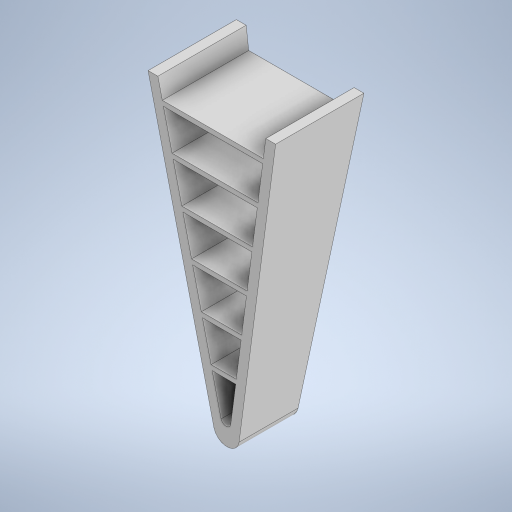
# Autodesk Inventor part: finley_gripper_60
Saved by Autodesk Inventor 2024 (Build 280153000, 153)
## iProperties
Created: 2024-09-23
Part Number: finley_gripper_60
Material: 一般
Document SubType Name: Modeling
Designer: 1412z
Density: 1 g/cm^3
Appearance: 既定
Author: 1412z
Autodesk Inventor part; units mm, degrees
ref_plane "YZ Plane" through (0, 0, 0) normal (1, 0, 0) x (0, 1, 0)
ref_plane "XZ Plane" through (0, 0, 0) normal (0, 1, 0) x (-1, 0, 0)
ref_plane "XY Plane" through (0, 0, 0) normal (0, 0, 1) x (1, 0, 0)
sketch "スケッチ1" plane through (0, 0, 0) normal (0, 0, 1) x (1, 0, 0)
  line L0 (0, 0) -> (-26, 0)
  line L1 (0, 0) -> (-13, -73.8647)
  line L2 (-13, -73.8647) -> (-26, 0)
  dimension "d0" = 26
  dimension "d1" = 75
  constraints: 6 end point, 1 horizontal
  measures "d0" distance of L0.start L0.end
  measures "d1" distance of L0.start L1.end
extrude "押し出し1" add sketch "スケッチ1" along normal mid plane 18
sketch "スケッチ2" plane through (0, 0, 9) normal (0, 0, 1) x (1, 0, 0)
  line L0 (-26, 0) -> (0, 0) projected
  line L1 (-2, 0) -> (-24, 0)
  line L2 (-2, 0) -> (-12.9991, -62.5063)
  line L3 (-2, 0) -> (61.4667, 0) construction
  line L4 (-12.9991, -62.5063) -> (-24, 0)
  line L5 (-13, -73.8647) -> (-26, 0) projected
  point P0 (-15.5606, -59.3154)
  dimension "d5" = 22
  dimension "d6" = 99.98
  constraints: 8 end point, 2 point on line, 1 equal length, 1 horizontal, 1 parallel
  measures "d5" distance of L1.start L1.end
  measures "d6" angle of L2 L3
extrude "押し出し2" cut sketch "スケッチ2" against normal blind 20
fillet "フィレット2" radius 1 1 edges at (-12.9991, -62.5063, 0)
fillet "フィレット3" radius 2.6 1 edges at (-13, -73.8647, 0)
sketch "スケッチ3" plane through (0, 0, 9) normal (0, 0, 1) x (1, 0, 0)
  line L0 (-12.0143, -56.9099) -> (-2, 0) projected
  line L1 (-2.7039, -4) -> (-23.296, -4)
  line L2 (-13.984, -56.9099) -> (-24, 0) projected
  line L3 (-23.296, -4) -> (-23.296, -5)
  line L4 (-23.296, -5) -> (-2.7039, -5)
  line L5 (-2.7039, -5) -> (-2.7039, -4)
  point P0 (0, 0)
  point P1 (-23.12, -5)
  point P2 (-2.8798, -5)
  dimension "d11" = 1
  constraints: 8 end point, 3 perpendicular, 2 point on line, 1 horizontal
  measures "d11" distance of L1.end L3.end
extrude "押し出し3" add sketch "スケッチ3" against normal blind 18 contours L4 L2 L1 L0
sketch "スケッチ4" plane through (0, 0, 9) normal (0, 0, 1) x (1, 0, 0)
  line L0 (-3.119, -13.78) -> (-22.8808, -13.78)
  line L1 (-22.8808, -13.78) -> (-22.8808, -12.78)
  line L2 (-22.8808, -12.78) -> (-3.119, -12.78)
  line L3 (-3.119, -12.78) -> (-3.119, -13.78)
  line L4 (-3.119, -13.78) -> (-22.8808, -12.78) construction
  line L5 (-22.8808, -13.78) -> (-3.119, -12.78) construction
  line L6 (-5.0044, -22.56) -> (-20.9954, -22.56)
  line L7 (-20.9954, -22.56) -> (-20.9954, -21.56)
  line L8 (-20.9954, -21.56) -> (-5.0044, -21.56)
  line L9 (-5.0044, -21.56) -> (-5.0044, -22.56)
  line L10 (-5.0044, -22.56) -> (-20.9954, -21.56) construction
  line L11 (-20.9954, -22.56) -> (-5.0044, -21.56) construction
  line L12 (-6.4483, -31.34) -> (-19.5515, -31.34)
  line L13 (-19.5515, -31.34) -> (-19.5515, -30.34)
  line L14 (-19.5515, -30.34) -> (-6.4483, -30.34)
  line L15 (-6.4483, -30.34) -> (-6.4483, -31.34)
  line L16 (-6.4483, -31.34) -> (-19.5515, -30.34) construction
  line L17 (-19.5515, -31.34) -> (-6.4483, -30.34) construction
  line L18 (-7.4478, -40.12) -> (-18.552, -40.12)
  line L19 (-18.552, -40.12) -> (-18.552, -39.12)
  line L20 (-18.552, -39.12) -> (-7.4478, -39.12)
  line L21 (-7.4478, -39.12) -> (-7.4478, -40.12)
  line L22 (-7.4478, -40.12) -> (-18.552, -39.12) construction
  line L23 (-18.552, -40.12) -> (-7.4478, -39.12) construction
  line L24 (-9.5376, -48.9) -> (-16.4622, -48.9)
  line L25 (-16.4622, -48.9) -> (-16.4622, -47.9)
  line L26 (-16.4622, -47.9) -> (-9.5376, -47.9)
  line L27 (-9.5376, -47.9) -> (-9.5376, -48.9)
  line L28 (-9.5376, -48.9) -> (-16.4622, -47.9) construction
  line L29 (-16.4622, -48.9) -> (-9.5376, -47.9) construction
  point P0 (0, 0)
  point P1 (-12.9999, -13.28)
  point P2 (-12.9999, -22.06)
  point P3 (-12.9999, -30.84)
  point P4 (-12.9999, -39.62)
  point P5 (-12.9999, -48.4)
  dimension "d14" = 1
  dimension "d15" = 1
  dimension "d16" = 1
  dimension "d17" = 1
  dimension "d18" = 1
  constraints: 60 end point, 10 midpoint, 10 parallel, 5 horizontal, 5 perpendicular
  measures "d14" distance of L0.end L1.end
  measures "d15" distance of L6.end L7.end
  measures "d16" distance of L12.end L13.end
  measures "d17" distance of L18.end L19.end
  measures "d18" distance of L24.end L25.end
extrude "押し出し4" add sketch "スケッチ4" against normal blind 18
sketch "スケッチ5" plane through (0, 0, 0) normal (1, 0, 0) x (0, 1, 0)
  line L0 (-61.4647, -9) -> (-61.4647, 9) projected
  line L1 (-61.4647, 5.9) -> (-61.4647, 9)
  line L2 (0, 9) -> (-59.3154, 9) projected
  line L3 (-61.4647, 5.9) -> (0, 9)
  line L4 (0, 9) -> (-61.4647, 9)
  line L5 (-59.3154, -9) -> (-61.4647, -9) projected
  line L6 (-61.4647, -5.9) -> (-61.4647, -9)
  line L7 (-61.4647, -9) -> (0, -9)
  line L8 (0, -9) -> (-61.4647, -5.9)
  point P0 (0, 0)
  constraints: 12 end point, 3 point on line, 2 perpendicular, 1 collinear
extrude "押し出し5" cut sketch "スケッチ5" against normal blind 30
